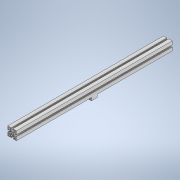
# Autodesk Inventor part: cross_AL_profile
Saved by Autodesk Inventor 2020 (Build 240168000, 168)
## iProperties
Created: 2022-07-15
Part Number: cross_AL_profile
Material: 일반
Document SubType Name: Modeling
Designer: SeungJin
Density: 1 g/cm^3
Appearance: 기본값
Author: SeungJin
Autodesk Inventor part; units mm, degrees
ref_plane "YZ Plane" through (0, 0, 0) normal (1, 0, 0) x (0, 1, 0)
ref_plane "XZ Plane" through (0, 0, 0) normal (0, 1, 0) x (-1, 0, 0)
ref_plane "XY Plane" through (0, 0, 0) normal (0, 0, 1) x (1, 0, 0)
sketch "스케치1" plane through (0, 0, 0) normal (0, 0, 1) x (1, 0, 0)
  line L0 (-15, 15) -> (15, 15)
  line L1 (15, 15) -> (-15, 15)
  line L2 (-15, 15) -> (-15, -15)
  line L3 (-15, -15) -> (15, -15)
  line L4 (15, -15) -> (15, 15)
  line L5 (-15, -15) -> (-5, -15)
  line L6 (-5, -15) -> (-5, -5)
  line L7 (-5, -5) -> (-15, -5)
  line L8 (-15, -5) -> (-15, -15)
  line L9 (-15, 15) -> (-5, 15)
  line L10 (-5, 15) -> (-5, 5)
  line L11 (-5, 5) -> (-15, 5)
  line L12 (-15, 5) -> (-15, 15)
  line L13 (15, -15) -> (5, -15)
  line L14 (5, -15) -> (5, -5)
  line L15 (5, -5) -> (15, -5)
  line L16 (15, -5) -> (15, -15)
  line L17 (15, 15) -> (5, 15)
  line L18 (5, 15) -> (5, 5)
  line L19 (5, 5) -> (15, 5)
  line L20 (15, 5) -> (15, 15)
  line L21 (-13, -7) -> (-7, -7)
  line L22 (-7, -7) -> (-7, -13)
  line L23 (-7, -13) -> (-13, -13)
  line L24 (-13, -13) -> (-13, -7)
  line L25 (-13, 7) -> (-7, 7)
  line L26 (-7, 7) -> (-7, 13)
  line L27 (-7, 13) -> (-13, 13)
  line L28 (-13, 13) -> (-13, 7)
  line L29 (7, -7) -> (7, -13)
  line L30 (7, -13) -> (13, -13)
  line L31 (13, -13) -> (13, -7)
  line L32 (13, -7) -> (7, -7)
  line L33 (7, 7) -> (7, 13)
  line L34 (7, 13) -> (13, 13)
  line L35 (13, 13) -> (13, 7)
  line L36 (13, 7) -> (7, 7)
  line L37 (-5, -15) -> (-3, -15)
  line L38 (-3, -15) -> (-3, -13)
  line L39 (-3, -13) -> (-5, -13)
  line L40 (-5, -13) -> (-5, -15)
  line L41 (5, -15) -> (3, -15)
  line L42 (3, -15) -> (3, -13)
  line L43 (3, -13) -> (5, -13)
  line L44 (5, -13) -> (5, -15)
  line L45 (5, 15) -> (3, 15)
  line L46 (3, 15) -> (3, 13)
  line L47 (3, 13) -> (5, 13)
  line L48 (5, 13) -> (5, 15)
  line L49 (-5, 15) -> (-3, 15)
  line L50 (-3, 15) -> (-3, 13)
  line L51 (-3, 13) -> (-5, 13)
  line L52 (-5, 13) -> (-5, 15)
  line L53 (15, -5) -> (13, -5)
  line L54 (13, -5) -> (13, -3)
  line L55 (13, -3) -> (15, -3)
  line L56 (15, -3) -> (15, -5)
  line L57 (15, 5) -> (13, 5)
  line L58 (13, 5) -> (13, 3)
  line L59 (13, 3) -> (15, 3)
  line L60 (15, 3) -> (15, 5)
  line L61 (-15, -5) -> (-13, -5)
  line L62 (-13, -5) -> (-13, -3)
  line L63 (-13, -3) -> (-15, -3)
  line L64 (-15, -3) -> (-15, -5)
  line L65 (-15, 5) -> (-13, 5)
  line L66 (-13, 5) -> (-13, 3)
  line L67 (-13, 3) -> (-15, 3)
  line L68 (-15, 3) -> (-15, 5)
  line L69 (5, -5) -> (-5, -5)
  line L70 (-5, -5) -> (-5, 5)
  line L71 (-5, 5) -> (5, 5)
  line L72 (5, 5) -> (5, -5)
  line L73 (5, -5) -> (-5, 5) construction
  line L74 (-5, -5) -> (5, 5) construction
  line L75 (-3.5858, -5) -> (-5, -3.5858)
  line L76 (-5, -3.5858) -> (-6.4142, -5)
  line L77 (-6.4142, -5) -> (-5, -6.4142)
  line L78 (-5, -6.4142) -> (-3.5858, -5)
  line L79 (-3.5858, -5) -> (-6.4142, -5) construction
  line L80 (-5, -3.5858) -> (-5, -6.4142) construction
  line L81 (-3.5858, 5) -> (-5, 6.4142)
  line L82 (-5, 6.4142) -> (-6.4142, 5)
  line L83 (-6.4142, 5) -> (-5, 3.5858)
  line L84 (-5, 3.5858) -> (-3.5858, 5)
  line L85 (-3.5858, 5) -> (-6.4142, 5) construction
  line L86 (-5, 6.4142) -> (-5, 3.5858) construction
  line L87 (5, 3.5858) -> (6.4142, 5)
  line L88 (6.4142, 5) -> (5, 6.4142)
  line L89 (5, 6.4142) -> (3.5858, 5)
  line L90 (3.5858, 5) -> (5, 3.5858)
  line L91 (5, 3.5858) -> (5, 6.4142) construction
  line L92 (6.4142, 5) -> (3.5858, 5) construction
  line L93 (5, -3.5858) -> (6.4142, -5)
  line L94 (6.4142, -5) -> (5, -6.4142)
  line L95 (5, -6.4142) -> (3.5858, -5)
  line L96 (3.5858, -5) -> (5, -3.5858)
  line L97 (5, -3.5858) -> (5, -6.4142) construction
  line L98 (6.4142, -5) -> (3.5858, -5) construction
  line L99 (3, 3) -> (-3, 3)
  line L100 (-3, 3) -> (-3, -3)
  line L101 (-3, -3) -> (3, -3)
  line L102 (3, -3) -> (3, 3)
  point P0 (0, 0)
  point P1 (0, 0)
  point P2 (-10, 162)
  point P3 (-10, 162)
  point P4 (-10, 162)
  point P5 (-10, 162)
  point P6 (-18, 162)
  point P7 (-8, 152)
  point P8 (-10, 154)
  point P9 (0, 172)
  point P10 (0, 172)
  point P11 (0, 172)
  point P12 (0, 172)
  point P13 (8, 172)
  point P14 (10, 170)
  point P15 (-2, 182)
  point P16 (0, 180)
  point P17 (0, 162)
  point P18 (0, 162)
  point P19 (0, 162)
  point P20 (0, 162)
  point P21 (8, 162)
  point P22 (0, 154)
  point P23 (-2, 152)
  point P24 (10, 164)
  point P25 (-18, 172)
  point P26 (-10, 180)
  point P27 (-8, 182)
  point P28 (1.4142, 162)
  point P29 (0, 163.4142)
  point P30 (-1.4142, 162)
  point P31 (0, 160.5858)
  point P32 (0, 173.4142)
  point P33 (-1.4142, 172)
  point P34 (0, 170.5858)
  point P35 (1.4142, 172)
  point P36 (-11.4142, 172)
  point P37 (-10, 170.5858)
  point P38 (-8.5858, 172)
  point P39 (-10, 173.4142)
  point P40 (-10, 160.5858)
  point P41 (-8.5858, 162)
  point P42 (-10, 163.4142)
  point P43 (-11.4142, 162)
  point P44 (-18, 162)
  point P45 (-20, 162)
  point P46 (-10, 152)
  point P47 (-20, 182)
  point P48 (-20, 164)
  point P49 (-20, 164)
  point P50 (-20, 162)
  point P51 (-20, 170)
  point P52 (0, 0)
  point P53 (5, 15)
  dimension "d0" = 30
  dimension "d1" = 10
  dimension "d2" = 10
  dimension "d3" = 10
  dimension "d4" = 10
  dimension "d5" = 10
  dimension "d6" = 10
  dimension "d7" = 10
  dimension "d8" = 10
  dimension "d9" = 2
  dimension "d10" = 2
  dimension "d11" = 2
  dimension "d12" = 2
  dimension "d13" = 2
  dimension "d14" = 2
  dimension "d15" = 2
  dimension "d16" = 2
  dimension "d17" = 2
  dimension "d18" = 2
  dimension "d19" = 2
  dimension "d20" = 2
  dimension "d21" = 2
  dimension "d22" = 2
  dimension "d23" = 2
  dimension "d24" = 2
  dimension "d25" = 2
  dimension "d26" = 2
  dimension "d27" = 2
  dimension "d28" = 2
  dimension "d29" = 2
  dimension "d30" = 2
  dimension "d31" = 2
  dimension "d32" = 2
  dimension "d33" = 2
  dimension "d34" = 2
  dimension "d35" = 2
  dimension "d36" = 2
  dimension "d37" = 2
  constraints: 206 end point, 48 parallel, 23 perpendicular, 15 horizontal, 11 midpoint, 1 coincident, 15 other
  measures "d0" distance of L5.start L1.end
  measures "d1" distance of L61.start L7.start
  measures "d2" distance of L7.start L5.end
  measures "d3" distance of L10.end L11.end
  measures "d4" distance of L52.end L10.end
  measures "d5" distance of L14.end L15.end
  measures "d6" distance of L13.end L14.end
  measures "d7" distance of L57.start L19.start
  measures "d8" distance of L19.start L17.end
  measures "d9" distance between parallel lines of L7 L21
  measures "d10" distance between parallel lines of L11 L25
  measures "d11" distance between parallel lines of L14 L29
  measures "d12" distance between parallel lines of L18 L33
  measures "d13" distance of L39.end L38.end
  measures "d14" distance of L38.end L38.start
  measures "d15" distance of L43.start L43.end
  measures "d16" distance of L41.end L43.start
  measures "d17" distance of L48.start L46.end
  measures "d18" distance of L46.end L46.start
  measures "d19" distance of L51.start L51.end
  measures "d20" distance of L50.start L51.start
  measures "d21" distance of L55.start L55.end
  measures "d22" distance of L54.start L55.start
  measures "d23" distance of L59.end L58.end
  measures "d24" distance of L58.end L58.start
  measures "d25" distance of L63.end L63.start
  measures "d26" distance of L63.start L62.start
  measures "d27" distance of L66.end L68.start
  measures "d28" distance of L66.start L66.end
  measures "d29" distance of L78.end L80.start
  measures "d30" distance of L77.start L80.start
  measures "d31" distance of L81.start L81.end
  measures "d32" distance of L82.end L81.end
  measures "d33" distance of L87.start L87.end
  measures "d34" distance of L91.end L87.end
  measures "d35" distance of L96.end L93.end
  measures "d36" distance of L93.end L97.end
  measures "d37" distance between parallel lines of L71 L99
extrude "돌출1" add sketch "스케치1" against normal blind 540 contours L0 L10 L82 L11 L2 | L0 L50 L51 L10 | L11 L66 L67 L2 | L0 L18 L47 L46 | L81 L71 L10 | L10 L11 L82 | L63 L62 L7 L2 | L11 L70 L83 | L0 L4 L19 L88 L18 | L71 L84 L70 | L71 L90 L72 L96 L69 L75 L70 L84 | L7 L77 L6 L3 L2 | L89 L18 L71 | L71 L72 L90 | L75 L69 L70 | L70 L7 L76 | L4 L59 L58 L19 | L88 L19 L18 | L19 L87 L72 | L6 L39 L38 L3 | L7 L6 L77 | L69 L78 L6 | L93 L15 L72 | L72 L69 L96 | L69 L14 L95 | L4 L15 L54 L55 | L15 L94 L14 | L15 L4 L3 L14 L94 | L42 L43 L14 L3
sketch "스케치2" plane through (3, -15, 0) normal (0, -1, 0) x (1, 0, 0)
  line L0 (12, 0) -> (12, -540) projected
  line L1 (-18, 0) -> (-18, -540) projected
  line L2 (-18, 0) -> (-6, 0) projected
  line L3 (0, 0) -> (12, 0) projected
  line L4 (-6, -540) -> (-18, -540) projected
  line L5 (12, -540) -> (0, -540) projected
  line L6 (0.5858, -540) -> (-6.5858, -540) projected
  line L7 (-6.5858, 0) -> (0.5858, 0) projected
  line L8 (-18, 0) -> (-18, -540) projected
  line L9 (12, -260) -> (-18, -260)
  line L10 (-18, -260) -> (-18, -280)
  line L11 (-18, -280) -> (12, -280)
  line L12 (12, -280) -> (12, -260)
  line L13 (12, -260) -> (-18, -280) construction
  line L14 (-18, -260) -> (12, -280) construction
  point P0 (-3, 0)
  point P1 (-3, -270)
  point P2 (-3, -270)
  point P3 (12, -270)
  dimension "d192" = 20
  constraints: 12 end point, 4 midpoint, 2 parallel, 1 horizontal, 1 horizontal alignment, 1 perpendicular, 1 point on line
  measures "d192" distance of L10.end L9.end
extrude "돌출2" add sketch "스케치2" along normal blind 10 contours L0 L11 L1 L9
